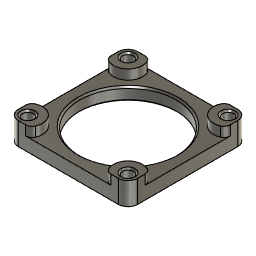
nema-17-mt-mount (Autodesk Fusion 360 design; units mm, degrees)
Autodesk Fusion 360 part; units mm, degrees
sketch "Sketch1" plane through (0, 0, 0) normal (0, 0, 1) x (1, 0, 0)
  line L0 (18.5, 18.5) -> (-18.5, 18.5)
  line L1 (-18.5, 18.5) -> (-18.5, -18.5)
  line L2 (-18.5, -18.5) -> (18.5, -18.5)
  line L3 (18.5, -18.5) -> (18.5, 18.5)
  line L4 (18.5, 18.5) -> (-18.5, -18.5) construction
  line L5 (-18.5, 18.5) -> (18.5, -18.5) construction
  line L6 (-15.5, 15.5) -> (15.5, 15.5) construction
  line L7 (15.5, 15.5) -> (15.5, -15.5) construction
  line L8 (15.5, -15.5) -> (-15.5, -15.5) construction
  line L9 (-15.5, -15.5) -> (-15.5, 15.5) construction
  circle A0 centre (15.5, 15.5) radius 1.7
  circle A1 centre (-15.5, 15.5) radius 1.7
  circle A2 centre (-15.5, -15.5) radius 1.7
  circle A3 centre (15.5, -15.5) radius 1.7
  circle A4 centre (-15.5, 15.5) radius 4.5
  circle A5 centre (15.5, 15.5) radius 4.5
  circle A6 centre (15.5, -15.5) radius 4.5
  circle A7 centre (-15.5, -15.5) radius 4.5
  circle A8 centre (0, 0) radius 15
  circle A9 centre (0, 0) radius 2.5
  circle A10 centre (0, 0) radius 4
  circle A11 centre (0, 0) radius 6.5
  dimension "d1" = 31
  dimension "d2" = 37
  dimension "d3" = 3.4
  dimension "d4" = 3
  dimension "d5" = 9
  dimension "d6" = 30
  dimension "d7" = 5
  dimension "d8" = 8
  dimension "d9" = 2.5
  constraint horizontal L0
  constraint perpendicular L0 L1
  constraint parallel L0 L2
  constraint parallel L1 L3
  constraint coincident L4 A8.centre
  constraint coincident L5 A8.centre
  constraint coincident A8.centre A9.centre
  constraint equal L0 L3
  constraint horizontal L6
  constraint vertical L7
  constraint horizontal L8
  constraint vertical L9
  constraint coincident L5 L7.end
  constraint coincident L5 L6.start
  constraint coincident L4 L6.end
  constraint equal A2 A3
  constraint equal A0 A3
  constraint equal A0 A1
  constraint coincident L6.end L7.start
  constraint coincident L6.start L9.end
  constraint coincident L8.end L9.start
  constraint coincident L7.end L8.start
  constraint concentric A1 A4
  constraint concentric A0 A5
  constraint concentric A3 A6
  constraint concentric A2 A7
  constraint equal A4 A7
  constraint equal A4 A5
  constraint equal A5 A6
  constraint concentric A8 A9
  constraint concentric A8 A11
  measures "d1" distance of L6.start L6.end
  measures "d2" distance of L0.start L0.end
  measures "d3" diameter of A0
  measures "d4" distance of L3 L6.end
  measures "d5" diameter of A5
  measures "d6" diameter of A8
  measures "d7" diameter of A9
  measures "d8" diameter of A10
  measures "d9" distance of A10 A11
extrude "Extrude1" add sketch "Sketch1" along normal blind 7 contours L0 L3 A5 | L0 L1 A4 | L2 L3 A6 | L1 L2 A7 picked at (15.3396, 18.0651) picked at (-15.3396, 18.0651) picked at (15.3396, -18.0651) picked at (-15.3396, -18.0651) makes body 1 at (-12.0055, 18.3353, 4.6667) makes body 2 at (18.3353, -12.0055, 2.3333) makes body 3 at (-11.8733, -18.164, 2.3333) makes body 4 at (18.164, 11.8733, 2.3333)
extrude "Extrude4" add sketch "Sketch1" along normal up to surface (4 mm away) contours L0 L1 L2 L3 A4 A5 A6 A7 bodies 2 1 3 4
chamfer "Chamfer4" distance 0.5 angle 45 2 edges at (-13.9849, 5.4242, 0) (-13.9849, -5.4242, 4) on bodies 2
fillet "Fillet1" radius 3 4 edges at (18.5, 18.5, 3.5) (18.5, -18.5, 3.5) (-18.5, -18.5, 3.5) (-18.5, 18.5, 3.5) on bodies 2
fillet "Fillet2" radius 2 8 edges at (12.1459, 18.5, 5.5) (18.5, 12.1459, 5.5) (-12.1459, 18.5, 5.5) (-18.5, 12.1459, 5.5) (-18.5, -12.1459, 5.5) (-12.1459, -18.5, 5.5) (12.1459, -18.5, 5.5) (18.5, -12.1459, 5.5) on bodies 2
chamfer "Chamfer5" distance 0.5 angle 45 8 edges at (-17.085, -14.8853, 7) (-17.085, 16.1147, 7) (13.915, 16.1147, 7) (13.915, -14.8853, 7) (13.915, -14.8853, 0) (-17.085, -14.8853, 0) (-17.085, 16.1147, 0) (13.915, 16.1147, 0) on bodies 1 2 3 4
named bodies: "md-bod"
